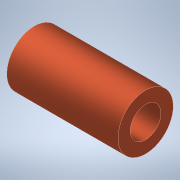
# Autodesk Inventor part: Spule
Saved by Autodesk Inventor 2021 (Build 250183000, 183)
## iProperties
Created: 2022-04-25
Part Number: Spule
Material: Kupfer
Document SubType Name: Modeling
Designer: Timo
Mass: 147.589 g
Surface Area: 58.3519 cm^2
Volume: 16.5088 cm^3
Density: 8.94 g/cm^3
Appearance: Kupfer - satiniert
Author: Timo
Autodesk Inventor part; units mm, degrees
ref_plane "YZ Plane" through (0, 0, 0) normal (1, 0, 0) x (0, 1, 0)
ref_plane "XZ Plane" through (0, 0, 0) normal (0, 1, 0) x (-1, 0, 0)
ref_plane "XY Plane" through (0, 0, 0) normal (0, 0, 1) x (1, 0, 0)
sketch "Skizze1" plane through (0, 0, 0) normal (0, 0, 1) x (1, 0, 0)
  line L0 (-21.75, 0) -> (21.75, 0)
  line L1 (-21.75, 6) -> (21.75, 6)
  line L2 (21.75, 6) -> (21.75, 10.8)
  line L3 (21.75, 10.8) -> (-21.75, 10.8)
  line L4 (-21.75, 10.8) -> (-21.75, 6)
  point P0 (0, 0)
  point P1 (0, 0)
  dimension "d0" = 43.5
  dimension "d1" = 12
  dimension "d4" = 4.8
  constraints: 10 end point, 3 perpendicular, 2 horizontal, 2 vertical alignment, 1 coincident, 1 midpoint
  measures "d0" distance of L0.start L0.end
  measures "d1" diameter of L1 L0
  measures "d4" distance between parallel lines of L3 L1
revolve "Umdrehung1" add sketch "Skizze1" angle 360 about axis through (-21.75, 0, 0) along (1, 0, 0)
